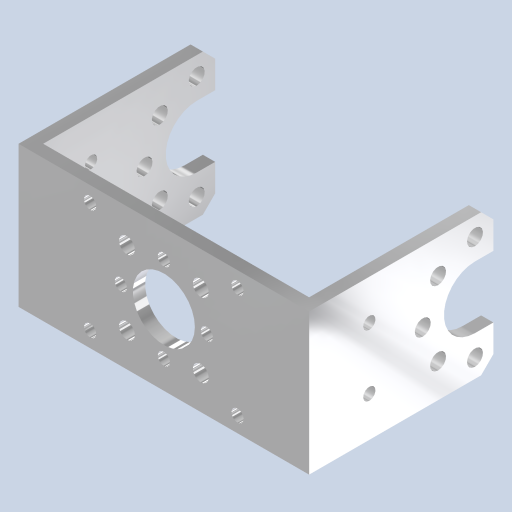
# Autodesk Inventor part: Servo_Arm
Saved by Autodesk Inventor 2023 (Build 270158000, 158)
## iProperties
Created: 2015-11-25
Part Number: Servo_Arm
Material: アルミニウム 5052
Document SubType Name: Modeling
Designer: hiroaki
Density: 2.68 g/cm^3
Appearance: アルミニウム - フラット
Mass: 10.9078 g
Surface Area: 50.5592 cm^2
Volume: 4.07007 cm^3
Author: hiroaki
Autodesk Inventor part; units mm, degrees
ref_plane "YZ Plane" through (0, 0, 0) normal (1, 0, 0) x (0, 1, 0)
ref_plane "XZ Plane" through (0, 0, 0) normal (0, 1, 0) x (-1, 0, 0)
ref_plane "XY Plane" through (0, 0, 0) normal (0, 0, 1) x (1, 0, 0)
sketch "スケッチ1" plane through (0, 0, 0) normal (0, 0, 1) x (1, 0, 0)
  line L0 (-23.65, 15) -> (-23.65, -15)
  line L1 (-23.65, -15) -> (23.65, -15)
  line L2 (23.65, -15) -> (23.65, 15)
  line L3 (23.65, 15) -> (21.65, 15)
  line L4 (21.65, 15) -> (21.65, -13)
  line L5 (21.65, -13) -> (-21.65, -13)
  line L6 (-21.65, -13) -> (-21.65, 15)
  line L7 (-21.65, 15) -> (-23.65, 15)
  point P0 (0, 0)
  point P1 (0, -13)
  point P2 (23.65, 0)
  dimension "d0" = 2
  dimension "d1" = 2
  dimension "d2" = 43.3
  dimension "d3" = 30
  constraints: 16 end point, 6 perpendicular, 2 equal length, 2 midpoint, 2 vertical, 1 horizontal alignment, 1 vertical alignment
  measures "d0" distance of L6.end L0.start
  measures "d1" distance between parallel lines of L5 L1
  measures "d2" distance of L4.end L5.end
  measures "d3" distance of L0.start L0.end
extrude "押し出し1" add sketch "スケッチ1" along normal blind 23
sketch "スケッチ2" plane through (23.65, -15, 0) normal (1, 0, 0) x (0, 0, -1)
  line L0 (0, 30) -> (-23, 30) projected
  line L1 (0, 0) -> (-23, 0) projected
  line L2 (-16.55, 31.0334) -> (-16.55, 27)
  arc A0 (-16.55, 27) -> (-6.45, 27) centre (-11.5, 27) ccw
  line L3 (-6.45, 27) -> (-6.45, 31.0334)
  line L4 (-6.45, 31.0334) -> (-16.55, 31.0334)
  circle A1 centre (-20, 27) radius 1.3
  circle A2 centre (-17.5104, 20.9896) radius 1.3
  circle A3 centre (-11.5, 18.5) radius 1.3
  circle A4 centre (-5.4896, 20.9896) radius 1.3
  circle A5 centre (-3, 27) radius 1.3
  circle A6 centre (-5.4896, 33.0104) radius 1.3
  circle A7 centre (-11.5, 35.5) radius 1.3
  circle A8 centre (-17.5104, 33.0104) radius 1.3
  circle A9 centre (-16.5, 9.8) radius 1
  line L5 (-11.5, 27) -> (-11.5, 30) construction
  circle A10 centre (-6.5, 9.8) radius 1
  point P0 (0, 15)
  dimension "d6" = 27
  dimension "d7" = 8.5
  dimension "d8" = 2.6
  dimension "d9" = 5.05
  dimension "d12" = 360
  dimension "d14" = 2
  dimension "d15" = 5
  dimension "d16" = 9.8
  constraints: 11 centre point, 8 end point, 3 vertical, 2 horizontal alignment, 2 point on circle, 1 midpoint, 1 perpendicular, 1 symmetric about line, 1 tangent, 1 vertical alignment, 18 other
  measures "d6" distance from line of L1 A1.centre
  measures "d7" distance of L5.start A1.centre
  measures "d8" diameter of A1
  measures "d9" radius of A0
  measures "d14" diameter of A9
  measures "d15" horizontal distance of A9.centre L5.start
  measures "d16" distance from line of L1 A9.centre
extrude "押し出し2" cut sketch "スケッチ2" against normal blind 100 contours L3 A0 L2 L0 | L0 L2 L4 L3 | A1 | A2 | A3 | A4 | A5 | A9 | A10
chamfer "面取り1" distance 2 angle 45 4 edges at (22.65, 15, 0) (22.65, 15, 23) (-22.65, 15, 23) (-22.65, 15, 0)
sketch "スケッチ3" plane through (-23.65, -15, 0) normal (0, -1, 0) x (1, 0, 0)
  line L0 (0, 23) -> (47.3, 23) projected
  line L1 (0, 0) -> (0, 23) projected
  circle A0 centre (23.65, 11.5) radius 5.05
  circle A1 centre (23.65, 18.5) radius 1
  circle A2 centre (17.6396, 17.5104) radius 1.3
  circle A3 centre (23.65, 11.5) radius 8.5 construction
  line L2 (23.65, 11.5) -> (17.6396, 17.5104) construction
  line L3 (23.65, 11.5) -> (23.65, 18.5) construction
  circle A4 centre (16.65, 11.5) radius 1
  circle A5 centre (17.6396, 5.4896) radius 1.3
  circle A6 centre (23.65, 4.5) radius 1
  circle A7 centre (29.6604, 5.4896) radius 1.3
  circle A8 centre (30.65, 11.5) radius 1
  circle A9 centre (29.6604, 17.5104) radius 1.3
  circle A10 centre (11.65, 2.5) radius 1
  line L4 (23.65, 11.5) -> (16.65, 11.5) construction
  circle A11 centre (11.65, 20.5) radius 1
  circle A12 centre (35.65, 2.5) radius 1
  circle A13 centre (35.65, 20.5) radius 1
  point P0 (23.65, 0)
  point P1 (0, 11.5)
  point P2 (23.65, 23)
  dimension "d25" = 17
  dimension "d22" = 10.1
  dimension "d23" = 2
  dimension "d24" = 7
  dimension "d26" = 2.6
  dimension "d27" = 45
  dimension "d30" = 360
  dimension "d32" = 2
  dimension "d33" = 9
  dimension "d34" = 12
  constraints: 13 centre point, 6 end point, 3 symmetric about line, 2 midpoint, 2 vertical alignment, 1 coincident, 1 horizontal, 1 horizontal alignment, 1 vertical, 23 other
  measures "d22" diameter of A0
  measures "d23" diameter of A1
  measures "d24" distance of L3.end A0.centre
  measures "d26" diameter of A2
  measures "d27" angle of L3 L2
  measures "d32" diameter of A10
  measures "d33" vertical distance of A0.centre A10.centre
  measures "d34" horizontal distance of A0.centre A10.centre
extrude "押し出し3" cut sketch "スケッチ3" against normal blind 10
equation "\"d1\" = d0"
